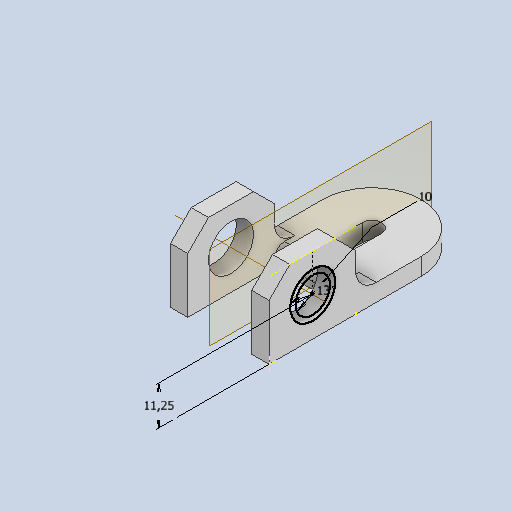
# Autodesk Inventor part: BeltDiscBottomPart
Saved by Autodesk Inventor 2022 (Build 260153000, 153)
## iProperties
Created: 2022-10-05
Part Number: BeltDiscBottomPart
Material: Generisch
Document SubType Name: Modeling
Designer: alexw
Density: 1 g/cm^3
Appearance: Vorgabe
Mass: 7.70089 g
Surface Area: 49.9228 cm^2
Volume: 7.70089 cm^3
Author: alexw
Autodesk Inventor part; units mm, degrees
ref_plane "YZ Plane" through (0, 0, 0) normal (1, 0, 0) x (0, 1, 0)
ref_plane "XZ Plane" through (0, 0, 0) normal (0, 1, 0) x (-1, 0, 0)
ref_plane "XY Plane" through (0, 0, 0) normal (0, 0, 1) x (1, 0, 0)
sketch "Skizze1" plane through (0, 0, 0) normal (0, 0, 1) x (1, 0, 0)
  line L0 (0, 0) -> (0, 22)
  line L1 (0, 22) -> (5, 22)
  line L2 (5, 22) -> (5, 5)
  line L3 (5, 5) -> (23.5, 5)
  line L4 (23.5, 5) -> (23.5, 22)
  line L5 (23.5, 22) -> (28.5, 22)
  line L6 (28.5, 22) -> (28.5, 0)
  line L7 (28.5, 0) -> (0, 0)
  line L8 (14.25, 5) -> (14.25, 0) construction
  line L9 (0, 11.55) -> (28.5, 11.55) construction
  dimension "d0" = 5
  dimension "d1" = 5
  dimension "d2" = 11.55
  dimension "d3" = 18.5
  dimension "d4" = 22
  dimension "d14" = 28.5
  constraints: 20 end point, 6 perpendicular, 4 point on line, 2 midpoint, 2 vertical, 1 collinear, 1 horizontal
  measures "d0" distance between parallel lines of L0 L2
  measures "d1" distance between parallel lines of L3 L7
  measures "d2" distance between parallel lines of L9 L7
  measures "d3" distance between parallel lines of L4 L2
  measures "d4" distance of L0.start L0.end
  measures "d14" distance between parallel lines of L6 L0
extrude "Extrusion1" add sketch "Skizze1" along normal blind 25
sketch "Skizze2" plane through (28.5, 0, 0) normal (1, 0, 0) x (0, 0, -1)
  circle A0 centre (-12.5, 11.25) radius 5
  line L0 (-12.5, 11.25) -> (-12.5, 22) construction
  line L1 (0, 22) -> (-25, 22) construction
  circle A1 centre (-12.5, 11.25) radius 6.5
  point P0 (0, 0)
  point P1 (-25, 0)
  dimension "d7" = 11.25
  dimension "d8" = 10
  dimension "d20" = 13
  constraints: 2 centre point, 2 end point, 1 coincident, 1 midpoint, 1 vertical
  measures "d7" vertical distance of L0.start point (-25, 0)
  measures "d8" diameter of A0
  measures "d20" diameter of A1
extrude "Extrusion2" cut sketch "Skizze2" against normal through all contours A0
sketch "Skizze3" plane through (5, 5, 0) normal (0, 1, 0) x (1, 0, 0)
  line L0 (18.5, -25) -> (0, -25) construction
  line L1 (9.25, -25) -> (9.25, 0) construction
  line L2 (18.5, 0) -> (0, 0) construction
  line L3 (9.25, -44.3) -> (9.25, -5.7) construction
  line L4 (18.5, -44.3) -> (18.5, -5.7)
  line L5 (0, -5.7) -> (0, -44.3)
  arc A0 (0, -44.3) -> (18.5, -44.3) centre (9.25, -44.3) ccw
  arc A1 (18.5, -5.7) -> (0, -5.7) centre (9.25, -5.7) ccw
  line L6 (29.2, -12.5) -> (-10.7, -12.5) construction
  line L7 (8, 0) -> (8, -25) construction
  line L8 (18, 0) -> (18, -25) construction
  line L9 (0, -25) -> (-5, -25) projected
  line L10 (9.25, 0) -> (1.9649, 0)
  line L11 (18.5, 0) -> (0, 0)
  line L12 (-5, 0) -> (23.5, 0) projected
  line L13 (18.5, 0) -> (18.5, -5.7)
  line L14 (0, 0) -> (0, -5.7)
  point P0 (16.5351, 0)
  dimension "d11" = 18.5
  dimension "d25" = 6.8
  dimension "d32" = 0.5
  dimension "d33" = 10
  constraints: 22 end point, 6 point on line, 5 point on circle, 4 tangent, 3 midpoint, 2 centre point, 2 perpendicular, 1 collinear, 1 parallel
  measures "d11" distance between parallel lines of L4 L5
  measures "d25" distance from line of L3.end L6
  measures "d32" distance between parallel lines of L4 L8
  measures "d33" distance between parallel lines of L7 L8
extrude "Extrusion3" cut sketch "Skizze3" against normal through all
sketch "Skizze4" plane through (5, 5, 0) normal (0, 1, 0) x (1, 0, 0)
  line L0 (18.5, 0) -> (0, 0) projected
  line L1 (9.25, -11) -> (9.25, 19) construction
  line L2 (-5, 0) -> (23.5, 0) projected
  line L3 (0, -11) -> (0, 19)
  line L4 (18.5, 19) -> (18.5, -11)
  arc A0 (0, -11) -> (18.5, -11) centre (9.25, -11) ccw
  arc A1 (18.5, 19) -> (0, 19) centre (9.25, 19) ccw
  line L5 (6.5, 19) -> (6.5, -11)
  arc A2 (6.5, -11) -> (12, -11) centre (9.25, -11) ccw
  line L6 (12, -11) -> (12, 19)
  arc A3 (12, 19) -> (6.5, 19) centre (9.25, 19) ccw
  arc A4 (6.5, 6.75) -> (12, 6.75) centre (9.25, 6.75) ccw
  line L7 (23.5, -11) -> (23.5, 19)
  arc A5 (23.5, 19) -> (-5, 19) centre (9.25, 19) ccw
  line L8 (-5, 19) -> (-5, -11)
  arc A6 (-5, -11) -> (23.5, -11) centre (9.25, -11) ccw
  arc A7 (18.5, 0) -> (0, 0) centre (9.25, -11.8084) ccw
  point P0 (9.25, 4)
  point P1 (18.5, 0)
  point P2 (6.5, 0)
  point P3 (12, 0)
  point P4 (8.25, 0)
  point P5 (9.25, 0)
  point P6 (18.5, -5.7)
  point P7 (0, -5.7)
  point P8 (0, -5.7)
  dimension "d15" = 15
  dimension "d18" = 5.5
  dimension "d26" = 4
  dimension "d34" = 5
  dimension "d35" = 15
  constraints: 17 point on circle, 16 end point, 8 centre point, 6 tangent, 4 point on line, 3 parallel, 2 midpoint, 1 perpendicular, 6 other
  measures "d15" distance of point (9.25, 4) L1.end
  measures "d18" distance between parallel lines of L6 L5
  measures "d26" distance from line of point (9.25, 4) L0
  measures "d34" distance between parallel lines of L4 L7
  measures "d35" radius of A7
extrude "Extrusion4" add sketch "Skizze4" against normal up to surface (5 mm away) contours L4 A1 L3 L2 L8 A5 L7 | A7 L6 A3 L5 L3 A1 L4 | L0 L6 A7 | L0 L5 A7 L6 | A7 L5 A4 L6 | L0 A7 L5
extrude "Extrusion5" cut sketch "Skizze2" against normal blind 5
extrude "Extrusion6" cut sketch "Skizze2" along normal blind 5 from surface at -28.5
chamfer "Fase1" distance 6 angle 45 4 edges at (26, 22, 25) (2.5, 22, 25) (2.5, 22, 0) (26, 22, 0)
fillet "Rundung4" radius 6 2 edges at (26, 5, 0) (2.5, 5, 0)
ref_plane "Arbeitsebene2" through (14.25, 0, -19) normal (1, 0, 0) x (0, 0, -1)
fillet "Rundung5" radius 3 1 edges at (14.25, 5, 0)
